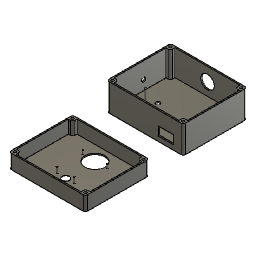
boitier v1 v4 (Autodesk Fusion 360 design; units mm, degrees)
Autodesk Fusion 360 part; units mm, degrees
sketch "Esquisse1" plane through (0, 0, 0) normal (0, 1, 0) x (1, 0, 0)
  arc A0 through (65, -26.5, 23.5) (64.1213, -26.5, 25.6213) (62, -26.5, 26.5)
  line L0 (65, -26.5, 23.5) -> (65, -26.5, -0.5)
  circle A1 through (4.9, -26.5, 0) (2.8, -26.5, 1.2124) (2.8, -26.5, -1.2124)
  circle A2 through (62.9, -26.5, 0) (60.8, -26.5, 1.2124) (60.8, -26.5, -1.2124)
  line L1 (3, -26.5, 26.5) -> (62, -26.5, 26.5)
  circle A3 through (62.9, -26.5, 23) (60.8, -26.5, 24.2124) (60.8, -26.5, 21.7876)
  circle A4 through (4.9, -26.5, 23) (2.8, -26.5, 24.2124) (2.8, -26.5, 21.7876)
  line L2 (62, -26.5, -3.5) -> (3, -26.5, -3.5)
  arc A5 through (62, -26.5, -3.5) (64.1213, -26.5, -2.6213) (65, -26.5, -0.5)
  arc A6 through (0, -26.5, -0.5) (0.8787, -26.5, -2.6213) (3, -26.5, -3.5)
  arc A7 through (3, -26.5, 26.5) (0.8787, -26.5, 25.6213) (0, -26.5, 23.5)
  line L3 (0, -26.5, -0.5) -> (0, -26.5, 23.5)
  point P0 (32.5, -26.5)
  point P1 (0, -26.5)
  point P2 (0, -26.5)
  point P3 (65, -26.5)
  point P4 (0, -26.5)
  point P5 (32.5, -26.5)
  dimension "d1" = 65
  dimension "d2" = 30
  dimension "d5" = 58
  dimension "d6" = 23
  dimension "d7" = 2.8
  dimension "d8" = 2.8
  dimension "d9" = 2.8
  dimension "d10" = 2.8
  dimension "d11" = 3
  constraint coincident P4 P2
  constraint coincident P5 P0
  measures "d1" distance of P4 P3
  measures "d2" distance of P4 P2
sketch "Esquisse2" plane through (0, 0, 0) normal (0, 0, 1) x (1, 0, 0)
  line L0 (-10, 65.4111) -> (75, 65.4111)
  line L1 (75, 65.4111) -> (75, -5)
  line L2 (75, -5) -> (-10, -5)
  line L3 (-10, -5) -> (-10, 65.4111)
  line L4 (-10, -5) -> (-5, -5)
  line L5 (-5, -5) -> (-5, 0)
  line L6 (-5, 0) -> (-10, 0)
  line L7 (-10, 0) -> (-10, -5)
  line L8 (75, -5) -> (70, -5)
  line L9 (70, -5) -> (70, 0)
  line L10 (70, 0) -> (75, 0)
  line L11 (75, 0) -> (75, -5)
  line L12 (-10, 65.4111) -> (-5, 65.4111)
  line L13 (-5, 65.4111) -> (-5, 60)
  line L14 (-5, 60) -> (-10, 60)
  line L15 (-10, 60) -> (-10, 65.4111)
  line L16 (75, 65.4111) -> (70, 65.4111)
  line L17 (70, 65.4111) -> (70, 60)
  line L18 (70, 60) -> (75, 60)
  line L19 (75, 60) -> (75, 65.4111)
  constraint horizontal L0
  constraint vertical L1
  constraint horizontal L2
  constraint vertical L3
  constraint horizontal L4
  constraint vertical L5
  constraint horizontal L6
  constraint vertical L7
  constraint horizontal L8
  constraint vertical L9
  constraint horizontal L10
  constraint vertical L11
  constraint horizontal L12
  constraint vertical L13
  constraint horizontal L14
  constraint vertical L15
  constraint horizontal L16
  constraint vertical L17
  constraint horizontal L18
  constraint vertical L19
extrude "Extrusion2" add sketch "Esquisse2" along normal blind 30 makes body 1
shell "Coque1" thickness 1.5 outward yes removed faces 1 at (20, 18.4704, 30) on bodies 1
extrude "Extrusion3" add sketch "Esquisse1" against normal blind 15 separate body contours A1 | A2 | A3 | A4 in plane through (0, 0, 26.5) normal (0, 0, -1) makes body 2 at (61.5349, 24.3996, 36.5) makes body 3 at (61.5349, 1.3996, 36.5) makes body 4 at (2.107, 22.8606, 36.5) makes body 5 at (2.107, -0.1394, 36.5)
move_face "DécalerLesFaces1" offset -0.25 4 faces at (2.107, 22.8606, 36.5) (61.5349, 24.3996, 36.5) (2.107, -0.1394, 36.5) (61.5349, 1.3996, 36.5) on bodies 2 3 4 5
move_body "Déplacer1" bodies 5 4 3 2 to x (1, 0, 0) y (0, 1, 0) z (0, 0, 1) at (0, 0, -27)
combine "Combiner1" operation add target body 1 tool bodies 4 5 2 3
sketch "Esquisse5" plane through (0, -6.5, 0) normal (0, -1, 0) x (1, 0, 0)
  line L0 (-11.5, -1.5) -> (76.5, -1.5)
  line L1 (76.5, -1.5) -> (76.5, 30)
  line L2 (76.5, 30) -> (-11.5, 30)
  line L3 (-11.5, 30) -> (-11.5, -1.5)
  line L4 (65, 27) -> (65, -6) construction
  line L5 (65, 4) -> (48, 4)
  line L6 (48, 4) -> (48, 14)
  line L7 (48, 14) -> (65, 14)
  line L8 (65, 14) -> (65, 4)
  dimension "d25" = 17
  dimension "d26" = 10
  constraint perpendicular L0 L4
  constraint horizontal L5
  constraint vertical L6
  constraint horizontal L7
  constraint vertical L8
  constraint coincident L4 L5.start
  measures "d25" distance of L5.start L5.end
  measures "d26" distance of L5.start L7.end
extrude "Extrusion4" cut sketch "Esquisse5" against normal blind 4 contours L5 L6 L7 L8 bodies 1
extrude "Extrusion5" add sketch "Esquisse2" along normal blind 30 contours L0 L3 L12 L13 L14 L15 | L0 L1 L16 L17 L18 L19 | L2 L3 L4 L5 L6 L7 | L1 L2 L8 L9 L10 L11 bodies 1
fillet "Congé1" radius 2.5 4 edges at (70, 60, 15) (70, 0, 15) (-5, 60, 15) (-5, 0, 15) on bodies 1
fillet "Congé2" radius 2.5 4 edges at (-11.5, 66.9111, 14.25) (76.5, 66.9111, 14.25) (-11.5, -6.5, 14.25) (76.5, -6.5, 14.25) on bodies 1
hole "Perçage1" at (-11.5, 34.3559, 11.1927) direction (1, 0, 0) diameter 5 depth 10 tip angle 118 bodies 1
hole "Perçage2" at (32.5, 66.9111, 14.25) direction (0, -1, 0) diameter 15.5 depth 10 tip angle 118 bodies 1
move_body "Déplacer2" bodies 1 to x (1, 0, 0) y (0, 1, 0) z (0, 0, 1) at (0, 0, 20)
extrude "Extrusion6" add sketch "Esquisse2" along normal blind 15 separate body makes body 6
shell "Coque2" thickness 1.5 outward yes removed faces 1 at (20, 18.4704, 0) on bodies 6
fillet "Congé3" radius 2.5 4 edges at (76.5, 66.9111, 8.25) (76.5, -6.5, 8.25) (-11.5, 66.9111, 8.25) (-11.5, -6.5, 8.25) on bodies 6
extrude "Extrusion7" add sketch "Esquisse2" along normal blind 15 contours L0 L3 L12 L13 L14 L15 | L0 L1 L16 L17 L18 L19 | L2 L3 L4 L5 L6 L7 | L1 L2 L8 L9 L10 L11 bodies 6
fillet "Congé4" radius 2.5 4 edges at (-5, 0, 7.5) (-5, 60, 7.5) (70, 60, 7.5) (70, 0, 7.5) on bodies 6
move_body "Déplacer3" bodies 1 to x (1, 0, 0) y (0, 1, 0) z (0, 0, 1) at (0, 0, -60)
sketch "Esquisse6" plane through (0, 0, 16.5) normal (0, 0, 1) x (1, 0, 0)
  arc A0 (-11.5, -4) -> (-9, -6.5) centre (-9, -4) ccw
  line L0 (-9, -6.5) -> (74, -6.5)
  arc A1 (74, -6.5) -> (76.5, -4) centre (74, -4) ccw
  line L1 (76.5, -4) -> (76.5, 64.4111)
  arc A2 (76.5, 64.4111) -> (74, 66.9111) centre (74, 64.4111) ccw
  line L2 (74, 66.9111) -> (-9, 66.9111)
  arc A3 (-9, 66.9111) -> (-11.5, 64.4111) centre (-9, 64.4111) ccw
  line L3 (-11.5, 64.4111) -> (-11.5, -4)
  line L4 (-10.7678, 66.1789) -> (75.7678, -5.7678) construction
  line L5 (75.7678, 66.1789) -> (-10.7678, -5.7678) construction
  line L6 (32.5, 66.9111) -> (32.5, -6.5) construction
  line L7 (-11.5, 30.2055) -> (76.5, 30.2055) construction
  line L8 (76.5, 30.2055) -> (32.5, -6.5) construction
  line L9 (32.5, -6.5) -> (-11.5, 30.2055) construction
  line L10 (10.5, 48.5583) -> (76.5, 48.5583) construction
  line L11 (10.5, 48.5583) -> (-11.5, 48.5583) construction
  line L12 (10.5, 11.8528) -> (76.5, 11.8528) construction
  line L13 (10.5, 11.8528) -> (-11.5, 11.8528) construction
  circle A4 centre (32.5, 11.8528) radius 11.5 construction
  line L14 (18.5, 18.3528) -> (46.5, 18.3528) construction
  line L15 (46.5, 18.3528) -> (46.5, 5.3528) construction
  line L16 (46.5, 5.3528) -> (18.5, 5.3528) construction
  line L17 (18.5, 5.3528) -> (18.5, 18.3528) construction
  line L18 (18.5, 18.3528) -> (46.5, 5.3528) construction
  line L19 (46.5, 18.3528) -> (18.5, 5.3528) construction
  circle A5 centre (32.5, 11.8528) radius 11.5
  circle A6 centre (18.5, 11.8528) radius 0.75
  circle A7 centre (46.5, 11.8528) radius 0.75
  line L20 (44.5, 61.0583) -> (20.5, 61.0583)
  line L21 (20.5, 61.0583) -> (20.5, 36.0583)
  line L22 (20.5, 36.0583) -> (44.5, 36.0583)
  line L23 (44.5, 36.0583) -> (44.5, 61.0583)
  line L24 (44.5, 61.0583) -> (20.5, 36.0583) construction
  line L25 (20.5, 61.0583) -> (44.5, 36.0583) construction
  line L26 (20.5, 36.0583) -> (44.5, 36.0583) construction
  line L27 (44.5, 36.0583) -> (44.5, 45.5583) construction
  line L28 (44.5, 45.5583) -> (20.5, 45.5583) construction
  line L29 (20.5, 45.5583) -> (20.5, 36.0583) construction
  line L30 (28.45, 49.6083) -> (36.55, 49.6083)
  line L31 (36.55, 49.6083) -> (36.55, 41.5083)
  line L32 (36.55, 41.5083) -> (28.45, 41.5083)
  line L33 (28.45, 41.5083) -> (28.45, 49.6083)
  line L34 (28.45, 49.6083) -> (36.55, 41.5083) construction
  line L35 (36.55, 49.6083) -> (28.45, 41.5083) construction
  line L36 (20.5, 61.0583) -> (22.5, 61.0583) construction
  line L37 (22.5, 61.0583) -> (22.5, 59.0583) construction
  line L38 (22.5, 59.0583) -> (20.5, 59.0583) construction
  line L39 (20.5, 59.0583) -> (20.5, 61.0583) construction
  line L40 (44.5, 61.0583) -> (42.5, 61.0583) construction
  line L41 (42.5, 61.0583) -> (42.5, 59.0583) construction
  line L42 (42.5, 59.0583) -> (44.5, 59.0583) construction
  line L43 (44.5, 59.0583) -> (44.5, 61.0583) construction
  line L44 (20.5, 36.0583) -> (22.5, 36.0583) construction
  line L45 (20.5, 38.0583) -> (20.5, 36.0583) construction
  line L46 (44.5, 36.0583) -> (42.5, 36.0583) construction
  line L47 (44.5, 38.0583) -> (44.5, 36.0583) construction
  circle A8 centre (22.5, 59.0583) radius 0.9
  circle A9 centre (42.5, 59.0583) radius 0.9
  line L48 (22.5, 61.0583) -> (22.5, 36.0583) construction
  line L49 (42.5, 61.0583) -> (42.5, 36.0583) construction
  circle A10 centre (22.5, 45.5583) radius 0.9
  circle A11 centre (42.5, 45.5583) radius 0.9
  circle A12 centre (32.5, 45.5583) radius 4
  point P0 (32.5, 11.8528)
  point P1 (32.5, 48.5583)
  point P2 (32.5, 45.5583)
  dimension "d50" = 23
  dimension "d51" = 28
  dimension "d52" = 13
  dimension "d53" = 1.5
  dimension "d54" = 1.5
  dimension "d59" = 24
  dimension "d60" = 25
  dimension "d61" = 9.5
  dimension "d62" = 8.1
  dimension "d63" = 8.1
  dimension "d64" = 2
  dimension "d65" = 2
  dimension "d66" = 2
  dimension "d67" = 2
  dimension "d68" = 2
  dimension "d69" = 2
  dimension "d70" = 2
  dimension "d71" = 2
  dimension "d72" = 1.8
  dimension "d73" = 1.8
  dimension "d74" = 1.8
  dimension "d75" = 1.8
  dimension "d76" = 8
  constraint midpoint A3 L4.start
  constraint midpoint A1 L4.end
  constraint midpoint A2 L5.start
  constraint midpoint A0 L5.end
  constraint midpoint L2 L6.start
  constraint midpoint L0 L6.end
  constraint midpoint L3 L7.start
  constraint midpoint L1 L7.end
  constraint coincident L1 L10.end
  constraint perpendicular L1 L10
  constraint coincident L3 L11.end
  constraint perpendicular L3 L11
  constraint midpoint L9 L12.start
  constraint coincident L1 L12.end
  constraint perpendicular L1 L12
  constraint coincident L3 L13.end
  constraint perpendicular L3 L13
  constraint coincident L12 P0
  constraint coincident L6 P0
  constraint horizontal L14
  constraint perpendicular L14 L15
  constraint parallel L14 L16
  constraint parallel L15 L17
  constraint coincident L18 P0
  constraint coincident L19 P0
  constraint coincident P0 A4.centre
  constraint midpoint L17 A6.centre
  constraint midpoint L15 A7.centre
  constraint horizontal L20
  constraint perpendicular L20 L21
  constraint parallel L20 L22
  constraint parallel L21 L23
  constraint coincident L24 P1
  constraint coincident L25 P1
  constraint coincident L10 P1
  constraint coincident L6 P1
  constraint horizontal L26
  constraint vertical L27
  constraint horizontal L28
  constraint vertical L29
  constraint horizontal L30
  constraint perpendicular L30 L31
  constraint parallel L30 L32
  constraint parallel L31 L33
  constraint coincident L34 P2
  constraint coincident L35 P2
  constraint midpoint L28 P2
  constraint horizontal L36
  constraint vertical L37
  constraint horizontal L38
  constraint vertical L39
  constraint horizontal L40
  constraint vertical L41
  constraint horizontal L42
  constraint vertical L43
  constraint horizontal L44
  constraint vertical L45
  constraint horizontal L46
  constraint vertical L47
  constraint coincident L37.end L38.start
  constraint coincident L41.end L42.start
  constraint perpendicular L26 L49
  constraint coincident L28 A10.centre
  constraint coincident L48 A10.centre
  constraint coincident L49 A11.centre
  constraint coincident L28 A11.centre
  constraint coincident P2 A12.centre
  measures "d50" diameter of A4
  measures "d51" distance of L15.end L16.end
  measures "d52" distance of L14.end L15.end
  measures "d53" diameter of A6
  measures "d54" diameter of A7
  measures "d59" distance of L21.end L22.end
  measures "d60" distance of L20.end L21.end
  measures "d61" distance of L21.end L28.end
  measures "d62" distance of L31.end L32.end
  measures "d63" distance of L30.end L31.end
  measures "d64" distance of L20.end L36.end
  measures "d65" distance of L20.end L38.end
  measures "d66" distance of L20.start L40.end
  measures "d67" distance of L20.start L42.end
  measures "d68" distance of L21.end L44.end
  measures "d69" distance of L21.end L45.start
  measures "d70" distance of L22.end L46.end
  measures "d71" distance of L22.end L47.start
  measures "d72" diameter of A8
  measures "d73" diameter of A9
  measures "d74" diameter of A10
  measures "d75" diameter of A11
  measures "d76" diameter of A12
extrude "Extrusion8" add sketch "Esquisse6" against normal blind 6 separate body contours A6 | A7 makes body 7 at (18.1578, 11.1854, 12.5) makes body 8 at (46.7031, 12.5747, 12.5)
extrude "Extrusion9" cut sketch "Esquisse6" against normal blind 4 contours A5 bodies 6
combine "Combiner2" operation add target body 6 tool bodies 8 7
extrude "Extrusion10" cut sketch "Esquisse6" against normal blind 5 contours A12 bodies 6
chamfer "Chanfrein1" distance 3 distance2 1 1 edges at (28.7707, 47.0048, 16.5) measured on face at (-0.287, 25.7512, 16.5) on bodies 6
extrude "Extrusion11" add sketch "Esquisse6" against normal blind 8 contours A8 | A9 | A10 | A11 bodies 6
sketch "Esquisse7" plane through (0, 0, 0) normal (0, 0, -1) x (-1, 0, 0)
  arc A0 (-70, -2.5) -> (-72.5, 0) centre (-72.5, -2.5) ccw
  line L0 (-72.5, 0) -> (-75, 0)
  line L1 (-75, 0) -> (-75, 60)
  line L2 (-75, 60) -> (-72.5, 60)
  arc A1 (-72.5, 60) -> (-70, 62.5) centre (-72.5, 62.5) ccw
  line L3 (-70, 62.5) -> (-70, 65.4111)
  line L4 (-70, 65.4111) -> (5, 65.4111)
  line L5 (5, 65.4111) -> (5, 62.5)
  arc A2 (5, 62.5) -> (7.5, 60) centre (7.5, 62.5) ccw
  line L6 (7.5, 60) -> (10, 60)
  line L7 (10, 60) -> (10, 0)
  line L8 (10, 0) -> (7.5, 0)
  arc A3 (7.5, 0) -> (5, -2.5) centre (7.5, -2.5) ccw
  line L9 (5, -2.5) -> (5, -5)
  line L10 (5, -5) -> (-70, -5)
  line L11 (-70, -5) -> (-70, -2.5)
  arc A4 (9, -6.5) -> (11.5, -4) centre (9, -4) ccw
  line L12 (11.5, -4) -> (11.5, 64.4111)
  arc A5 (11.5, 64.4111) -> (9, 66.9111) centre (9, 64.4111) ccw
  line L13 (9, 66.9111) -> (-74, 66.9111)
  arc A6 (-74, 66.9111) -> (-76.5, 64.4111) centre (-74, 64.4111) ccw
  line L14 (-76.5, 64.4111) -> (-76.5, -4)
  arc A7 (-76.5, -4) -> (-74, -6.5) centre (-74, -4) ccw
  line L15 (-74, -6.5) -> (9, -6.5)
  line L16 (-70.7322, 60.7322) -> (-75.7678, 66.1789) construction
  line L17 (5.7322, 60.7322) -> (10.7678, 66.1789) construction
  line L18 (5.7322, -0.7322) -> (10.7678, -5.7678) construction
  line L19 (-70.7322, -0.7322) -> (-75.7678, -5.7678) construction
  circle A8 centre (-73.25, 63.4555) radius 1.45
  circle A9 centre (-73.25, 63.4555) radius 2.75
  circle A10 centre (8.25, 63.4555) radius 1.45
  circle A11 centre (8.25, 63.4555) radius 2.75
  circle A12 centre (-73.25, -3.25) radius 1.45
  circle A13 centre (-73.25, -3.25) radius 2.75
  circle A14 centre (8.25, -3.25) radius 1.45
  circle A15 centre (8.25, -3.25) radius 2.75
  dimension "d88" = 2.9
  dimension "d89" = 5.5
  dimension "d90" = 2.9
  dimension "d91" = 5.5
  dimension "d92" = 2.9
  dimension "d93" = 5.5
  dimension "d94" = 2.9
  dimension "d95" = 5.5
  constraint midpoint A1 L16.start
  constraint midpoint A6 L16.end
  constraint midpoint A2 L17.start
  constraint midpoint A5 L17.end
  constraint midpoint A3 L18.start
  constraint midpoint A4 L18.end
  constraint midpoint A0 L19.start
  constraint midpoint A7 L19.end
  constraint midpoint L16 A8.centre
  constraint concentric A8 A9
  constraint midpoint L17 A10.centre
  constraint concentric A10 A11
  constraint midpoint L19 A12.centre
  constraint concentric A12 A13
  constraint midpoint L18 A14.centre
  constraint concentric A14 A15
  measures "d88" diameter of A8
  measures "d89" diameter of A9
  measures "d90" diameter of A10
  measures "d91" diameter of A11
  measures "d92" diameter of A12
  measures "d93" diameter of A13
  measures "d94" diameter of A14
  measures "d95" diameter of A15
extrude "Extrusion12" cut sketch "Esquisse7" along normal blind 28 contours A8 | A10 | A12 | A14 bodies 1
extrude "Extrusion13" cut sketch "Esquisse7" against normal blind 30 contours A8 | A10 | A12 | A14 bodies 6
move_body "Déplacer4" bodies 6 to x (1, 0, 0) y (0, 1, 0) z (0, 0, 1) at (0, 0, -2)
extrude "Extrusion14" cut sketch "Esquisse7" against normal blind 20 contours A9 | A11 | A13 | A15 bodies 6
sketch "Esquisse8" plane through (0, 0, 14.5) normal (0, 0, 1) x (1, 0, 0)
  circle A0 centre (-8.25, -3.25) radius 2.75
  circle A1 centre (-8.25, 63.4555) radius 2.75
  circle A2 centre (73.25, 63.4555) radius 2.75
  circle A3 centre (73.25, -3.25) radius 2.75
  arc A4 (-11.5, -4) -> (-9, -6.5) centre (-9, -4) ccw
  line L0 (-9, -6.5) -> (74, -6.5)
  arc A5 (74, -6.5) -> (76.5, -4) centre (74, -4) ccw
  line L1 (76.5, -4) -> (76.5, 64.4111)
  arc A6 (76.5, 64.4111) -> (74, 66.9111) centre (74, 64.4111) ccw
  line L2 (74, 66.9111) -> (-9, 66.9111)
  arc A7 (-9, 66.9111) -> (-11.5, 64.4111) centre (-9, 64.4111) ccw
  line L3 (-11.5, 64.4111) -> (-11.5, -4)
  circle A8 centre (32.5, 11.8528) radius 11.5
  circle A9 centre (32.5, 45.5583) radius 7
  line L4 (-2.0048, 6.1275) -> (-2.0048, 5.8365)
  line L5 (-2.0048, 5.8365) -> (-1.211, 5.8365)
  line L6 (-1.211, 5.8365) -> (-1.211, 4.7781)
  line L7 (-1.211, 4.7781) -> (-4.3596, 4.7781)
  line L8 (-4.3596, 4.7781) -> (-4.3596, 6.2995)
  spline S0 degree 3 poles (-4.3596, 6.2995) (-4.3596, 7.1726) (-3.8966, 7.7282) (-3.169, 7.7282) knots 0 0 0 0 1 1 1 1
  spline S1 degree 3 poles (-3.169, 7.7282) (-2.7192, 7.7282) (-2.3752, 7.5166) (-2.1768, 7.1329) knots 0 0 0 0 1 1 1 1
  line L9 (-2.1768, 7.1329) -> (-1.211, 7.7944)
  line L10 (-1.211, 7.7944) -> (-1.211, 6.6567)
  line L11 (-1.211, 6.6567) -> (-2.0048, 6.1275)
  line L12 (-3.5394, 6.2333) -> (-3.5394, 5.8497)
  line L13 (-3.5394, 5.8497) -> (-2.7985, 5.8497)
  line L14 (-2.7985, 5.8497) -> (-2.7985, 6.2333)
  spline S2 degree 3 poles (-2.7985, 6.2333) (-2.7985, 6.5244) (-2.9441, 6.6699) (-3.169, 6.6699) knots 0 0 0 0 1 1 1 1
  spline S3 degree 3 poles (-3.169, 6.6699) (-3.3939, 6.6699) (-3.5394, 6.5244) (-3.5394, 6.2333) knots 0 0 0 0 1 1 1 1
  spline S4 degree 3 poles (-2.7853, 8.006) (-3.7378, 8.006) (-4.4257, 8.7601) (-4.4257, 9.7788) knots 0 0 0 0 1 1 1 1
  spline S5 degree 3 poles (-4.4257, 9.7788) (-4.4257, 10.7974) (-3.7378, 11.5515) (-2.7853, 11.5515) knots 0 0 0 0 1 1 1 1
  spline S6 degree 3 poles (-2.7853, 11.5515) (-1.8328, 11.5515) (-1.1449, 10.7974) (-1.1449, 9.7788) knots 0 0 0 0 1 1 1 1
  spline S7 degree 3 poles (-1.1449, 9.7788) (-1.1449, 8.7601) (-1.8328, 8.006) (-2.7853, 8.006) knots 0 0 0 0 1 1 1 1
  spline S8 degree 3 poles (-2.7853, 10.4931) (-3.2748, 10.4931) (-3.5658, 10.1756) (-3.5658, 9.792) knots 0 0 0 0 1 1 1 1
  spline S9 degree 3 poles (-3.5658, 9.792) (-3.5658, 9.4083) (-3.2748, 9.0908) (-2.7853, 9.0908) knots 0 0 0 0 1 1 1 1
  spline S10 degree 3 poles (-2.7853, 9.0908) (-2.2958, 9.0908) (-2.0048, 9.4083) (-2.0048, 9.792) knots 0 0 0 0 1 1 1 1
  spline S11 degree 3 poles (-2.0048, 9.792) (-2.0048, 10.1756) (-2.2958, 10.4931) (-2.7853, 10.4931) knots 0 0 0 0 1 1 1 1
  line L15 (-4.3596, 11.9483) -> (-4.3596, 13.4961)
  spline S12 degree 3 poles (-4.3596, 13.4961) (-4.3596, 14.5545) (-3.7643, 15.2689) (-2.7853, 15.2689) knots 0 0 0 0 1 1 1 1
  spline S13 degree 3 poles (-2.7853, 15.2689) (-1.8064, 15.2689) (-1.211, 14.5412) (-1.211, 13.4961) knots 0 0 0 0 1 1 1 1
  line L16 (-1.211, 13.4961) -> (-1.211, 11.9483)
  line L17 (-1.211, 11.9483) -> (-4.3596, 11.9483)
  spline S14 degree 3 poles (-2.0312, 13.4565) (-2.0312, 13.9063) (-2.2958, 14.2105) (-2.7721, 14.2105) knots 0 0 0 0 1 1 1 1
  spline S15 degree 3 poles (-2.7721, 14.2105) (-3.2483, 14.2105) (-3.5129, 13.9062) (-3.5129, 13.4565) knots 0 0 0 0 1 1 1 1
  line L18 (-3.5129, 13.4565) -> (-3.5129, 13.0067)
  line L19 (-3.5129, 13.0067) -> (-2.0312, 13.0067)
  line L20 (-2.0312, 13.0067) -> (-2.0312, 13.4565)
  spline S16 degree 3 poles (-2.7853, 15.5334) (-3.7378, 15.5334) (-4.4257, 16.2875) (-4.4257, 17.3061) knots 0 0 0 0 1 1 1 1
  spline S17 degree 3 poles (-4.4257, 17.3061) (-4.4257, 18.3248) (-3.7378, 19.0789) (-2.7853, 19.0789) knots 0 0 0 0 1 1 1 1
  spline S18 degree 3 poles (-2.7853, 19.0789) (-1.8328, 19.0789) (-1.1449, 18.3248) (-1.1449, 17.3061) knots 0 0 0 0 1 1 1 1
  spline S19 degree 3 poles (-1.1449, 17.3061) (-1.1449, 16.2875) (-1.8328, 15.5334) (-2.7853, 15.5334) knots 0 0 0 0 1 1 1 1
  spline S20 degree 3 poles (-2.7853, 18.0205) (-3.2748, 18.0205) (-3.5658, 17.703) (-3.5658, 17.3194) knots 0 0 0 0 1 1 1 1
  spline S21 degree 3 poles (-3.5658, 17.3194) (-3.5658, 16.9357) (-3.2748, 16.6182) (-2.7853, 16.6182) knots 0 0 0 0 1 1 1 1
  spline S22 degree 3 poles (-2.7853, 16.6182) (-2.2958, 16.6182) (-2.0048, 16.9357) (-2.0048, 17.3194) knots 0 0 0 0 1 1 1 1
  spline S23 degree 3 poles (-2.0048, 17.3194) (-2.0048, 17.703) (-2.2958, 18.0205) (-2.7853, 18.0205) knots 0 0 0 0 1 1 1 1
  spline S24 degree 3 poles (-2.7853, 19.3567) (-3.751, 19.3567) (-4.4257, 20.0975) (-4.4257, 21.1161) knots 0 0 0 0 1 1 1 1
  spline S25 degree 3 poles (-4.4257, 21.1161) (-4.4257, 21.7379) (-4.2008, 22.2142) (-3.7907, 22.5317) knots 0 0 0 0 1 1 1 1
  line L21 (-3.7907, 22.5317) -> (-3.1954, 21.857)
  spline S26 degree 3 poles (-3.1954, 21.857) (-3.4335, 21.6718) (-3.5658, 21.4469) (-3.5658, 21.1691) knots 0 0 0 0 1 1 1 1
  spline S27 degree 3 poles (-3.5658, 21.1691) (-3.5658, 20.7325) (-3.2616, 20.4282) (-2.7853, 20.4282) knots 0 0 0 0 1 1 1 1
  spline S28 degree 3 poles (-2.7853, 20.4282) (-2.3091, 20.4282) (-2.0048, 20.7193) (-2.0048, 21.1691) knots 0 0 0 0 1 1 1 1
  spline S29 degree 3 poles (-2.0048, 21.1691) (-2.0048, 21.4469) (-2.1371, 21.6718) (-2.3752, 21.857) knots 0 0 0 0 1 1 1 1
  line L22 (-2.3752, 21.857) -> (-1.7799, 22.5317)
  spline S30 degree 3 poles (-1.7799, 22.5317) (-1.3698, 22.2274) (-1.1449, 21.7379) (-1.1449, 21.1161) knots 0 0 0 0 1 1 1 1
  spline S31 degree 3 poles (-1.1449, 21.1161) (-1.1317, 20.0975) (-1.8196, 19.3567) (-2.7853, 19.3567) knots 0 0 0 0 1 1 1 1
  line L23 (-1.7534, 24.9261) -> (-1.7534, 23.7355)
  line L24 (-1.7534, 23.7355) -> (-1.211, 23.5239)
  line L25 (-1.211, 23.5239) -> (-1.211, 22.4391)
  line L26 (-1.211, 22.4391) -> (-4.3596, 23.8149)
  line L27 (-4.3596, 23.8149) -> (-4.3596, 24.86)
  line L28 (-4.3596, 24.86) -> (-1.211, 26.2358)
  line L29 (-1.211, 26.2358) -> (-1.211, 25.1378)
  line L30 (-1.211, 25.1378) -> (-1.7534, 24.9261)
  line L31 (-2.5207, 24.6351) -> (-3.3145, 24.3308)
  line L32 (-3.3145, 24.3308) -> (-2.5207, 24.0266)
  line L33 (-2.5207, 24.0266) -> (-2.5207, 24.6351)
  line L34 (-1.211, 29.2124) -> (-2.6398, 29.1992)
  line L35 (-2.6398, 29.1992) -> (-1.4889, 28.5112)
  line L36 (-1.4889, 28.5112) -> (-1.4889, 28.0615)
  line L37 (-1.4889, 28.0615) -> (-2.5869, 27.3735)
  line L38 (-2.5869, 27.3735) -> (-1.1978, 27.3735)
  line L39 (-1.1978, 27.3735) -> (-1.1978, 26.4078)
  line L40 (-1.1978, 26.4078) -> (-4.3596, 26.4078)
  line L41 (-4.3596, 26.4078) -> (-4.3596, 27.2809)
  line L42 (-4.3596, 27.2809) -> (-2.6795, 28.3128)
  line L43 (-2.6795, 28.3128) -> (-4.3596, 29.305)
  line L44 (-4.3596, 29.305) -> (-4.3596, 30.1781)
  line L45 (-4.3596, 30.1781) -> (-1.211, 30.1914)
  line L46 (-1.211, 30.1914) -> (-1.211, 29.2124)
  line L47 (-4.3596, 35.4036) -> (-1.211, 34.0675)
  line L48 (-1.211, 34.0675) -> (-1.211, 33.0224)
  line L49 (-1.211, 33.0224) -> (-4.3596, 31.6862)
  line L50 (-4.3596, 31.6862) -> (-4.3596, 32.824)
  line L51 (-4.3596, 32.824) -> (-2.5207, 33.578)
  line L52 (-2.5207, 33.578) -> (-4.3596, 34.3453)
  line L53 (-4.3596, 34.3453) -> (-4.3596, 35.4036)
  line L54 (-4.3596, 37.0838) -> (-1.211, 37.0838)
  line L55 (-1.211, 37.0838) -> (-1.211, 36.0254)
  line L56 (-1.211, 36.0254) -> (-3.5526, 36.0254)
  line L57 (-3.5526, 36.0254) -> (-3.5526, 35.483)
  line L58 (-3.5526, 35.483) -> (-4.3596, 35.483)
  line L59 (-4.3596, 35.483) -> (-4.3596, 37.0838)
  spline S32 degree 3 poles (-1.7534, 37.4277) (-2.0974, 37.4277) (-2.3355, 37.6791) (-2.3355, 38.023) knots 0 0 0 0 1 1 1 1
  spline S33 degree 3 poles (-2.3355, 38.023) (-2.3355, 38.3537) (-2.1106, 38.6183) (-1.7534, 38.6183) knots 0 0 0 0 1 1 1 1
  spline S34 degree 3 poles (-1.7534, 38.6183) (-1.4095, 38.6183) (-1.1714, 38.367) (-1.1714, 38.023) knots 0 0 0 0 1 1 1 1
  spline S35 degree 3 poles (-1.1714, 38.023) (-1.1581, 37.6923) (-1.4095, 37.4277) (-1.7534, 37.4277) knots 0 0 0 0 1 1 1 1
  spline S36 degree 3 poles (-2.7853, 38.7639) (-3.8304, 38.7639) (-4.4257, 39.3592) (-4.4257, 40.1926) knots 0 0 0 0 1 1 1 1
  spline S37 degree 3 poles (-4.4257, 40.1926) (-4.4257, 41.026) (-3.8172, 41.6214) (-2.7853, 41.6214) knots 0 0 0 0 1 1 1 1
  spline S38 degree 3 poles (-2.7853, 41.6214) (-1.7534, 41.6214) (-1.1449, 41.026) (-1.1449, 40.1926) knots 0 0 0 0 1 1 1 1
  spline S39 degree 3 poles (-1.1449, 40.1926) (-1.1449, 39.3592) (-1.7402, 38.7639) (-2.7853, 38.7639) knots 0 0 0 0 1 1 1 1
  spline S40 degree 3 poles (-2.7853, 40.5498) (-3.3939, 40.5498) (-3.5791, 40.391) (-3.5791, 40.1926) knots 0 0 0 0 1 1 1 1
  spline S41 degree 3 poles (-3.5791, 40.1926) (-3.5791, 39.9942) (-3.3939, 39.8354) (-2.7853, 39.8354) knots 0 0 0 0 1 1 1 1
  spline S42 degree 3 poles (-2.7853, 39.8354) (-2.1768, 39.8354) (-1.9916, 39.9942) (-1.9916, 40.1926) knots 0 0 0 0 1 1 1 1
  spline S43 degree 3 poles (-1.9916, 40.1926) (-1.9916, 40.391) (-2.1768, 40.5498) (-2.7853, 40.5498) knots 0 0 0 0 1 1 1 1
hole "Perçage3" at (10.7385, 30.0484, -40) direction (0, 0, -1) diameter 5 depth 10 tip angle 118 bodies 1
hole "Perçage4" at (52.8474, 30.0484, -40) direction (0, 0, -1) diameter 5 depth 10 tip angle 118 bodies 1
move_body "Déplacer5" bodies 1 to x (1, 0, 0) y (0, 0, -1) z (0, 1, 0) at (0, 35, -48)
move_body "Déplacer6" bodies 6 to x (1, 0, 0) y (0, 0, 1) z (0, -1, 0) at (0, 16.5, 4.5)
move_body "Déplacer7" bodies 1 to x (1, 0, 0) y (0, 1, 0) z (0, 0, 1) at (0, 6.5, 0)
move_body "Déplacer8" bodies 6 to x (1, 0, 0) y (0, 1, 0) z (0, 0, 1) at (0, -2, 0)
extrude "Extrusion15" [rolled back] along distance -30 taper angle 0
